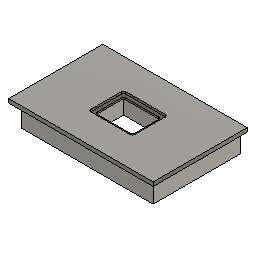
Freestafel - v1 v6 (Autodesk Fusion 360 design; units mm, degrees)
Autodesk Fusion 360 part; units mm, degrees
sketch "Sketch1" plane through (0, 0, 0) normal (0, 0, 1) x (1, 0, 0) in component "Freesblad"
  line L0 (0, 0) -> (660, 0)
  line L1 (660, 0) -> (660, 430)
  line L2 (660, 430) -> (0, 430)
  line L3 (0, 430) -> (0, 0)
  dimension "d10" = 660
  dimension "d11" = 430
  constraint horizontal L0
  constraint vertical L1
  constraint horizontal L2
  constraint vertical L3
  constraint coincident L0.start L3.end
  measures "d10" distance of L0.start L0.end
  measures "d11" distance of L0.start L2.end
extrude "Extrude1" add sketch "Sketch1" along normal blind 18 makes body 1 in component "Freesblad"
sketch "Sketch2" plane through (0, 0, 18) normal (0, 0, 1) x (-1, 0, 0) in component "Freesblad"
  line L0 (0, -430) -> (0, 0)
  line L1 (0, 0) -> (-660, 0)
  line L2 (-660, 0) -> (-660, -430)
  line L3 (-660, -430) -> (0, -430)
  line L4 (-420, -135) -> (-240, -135)
  line L5 (-230, -145) -> (-230, -285)
  line L6 (-240, -295) -> (-420, -295)
  line L7 (-430, -285) -> (-430, -145)
  line L8 (-430, -135) -> (-230, -295) construction
  line L9 (-230, -135) -> (-430, -295) construction
  arc A0 (-430, -285) -> (-420, -295) centre (-420, -285) ccw
  arc A1 (-240, -295) -> (-230, -285) centre (-240, -285) ccw
  arc A2 (-230, -145) -> (-240, -135) centre (-240, -145) ccw
  arc A3 (-420, -135) -> (-430, -145) centre (-420, -145) ccw
  arc A4 (-450, -285) -> (-420, -315) centre (-420, -285) ccw
  line L10 (-240, -315) -> (-420, -315)
  arc A5 (-240, -315) -> (-210, -285) centre (-240, -285) ccw
  line L11 (-210, -145) -> (-210, -285)
  arc A6 (-210, -145) -> (-240, -115) centre (-240, -145) ccw
  line L12 (-420, -115) -> (-240, -115)
  arc A7 (-420, -115) -> (-450, -145) centre (-420, -145) ccw
  line L13 (-450, -285) -> (-450, -145)
  point P0 (-330, -215)
  dimension "d16" = 200
  dimension "d17" = 160
  dimension "d18" = 10
  dimension "d19" = 10
  dimension "d20" = 10
  dimension "d21" = 10
  dimension "d40" = 215
  dimension "d41" = 330
  dimension "d42" = -20
  constraint horizontal L4
  constraint perpendicular L4 L5
  constraint parallel L4 L6
  constraint parallel L5 L7
  constraint coincident L8 P0
  constraint coincident L9 P0
  constraint coincident L9.end L6
  constraint coincident L9.end L7
  constraint tangent L6 A0
  constraint tangent L7 A0
  constraint coincident L8.end L5
  constraint coincident L8.end L6
  constraint tangent L5 A1
  constraint tangent L6 A1
  constraint coincident L9.start L5
  constraint coincident L9.start L4
  constraint tangent L5 A2
  constraint tangent L4 A2
  constraint coincident L8.start L7
  constraint coincident L8.start L4
  constraint tangent L7 A3
  constraint tangent L4 A3
  measures "d16" distance of L8.end L9.end
  measures "d17" distance of L9.start L8.end
  measures "d18" radius of A0
  measures "d19" radius of A1
  measures "d20" radius of A2
  measures "d21" radius of A3
  measures "d40" distance of L1 P0
  measures "d41" distance of L0 P0
  measures "d42" distance of A0
extrude "Extrude2" cut sketch "Sketch2" against normal blind 10 contours L4 L5 L6 L7 A0 A1 A2 A3 bodies 1 in component "Freesblad"
sketch "Sketch4" plane through (0, 0, 8) normal (0, 0, 1) x (-1, 0, 0) in component "Freesblad"
  arc A0 (-230, -145) -> (-240, -135) centre (-240, -145) ccw
  line L0 (-240, -135) -> (-420, -135)
  arc A1 (-420, -135) -> (-430, -145) centre (-420, -145) ccw
  line L1 (-430, -145) -> (-430, -285)
  arc A2 (-430, -285) -> (-420, -295) centre (-420, -285) ccw
  line L2 (-420, -295) -> (-240, -295)
  arc A3 (-240, -295) -> (-230, -285) centre (-240, -285) ccw
  line L3 (-230, -285) -> (-230, -145)
  line L4 (-245, -270) -> (-245, -160)
  line L5 (-255, -150) -> (-405, -150)
  line L6 (-415, -160) -> (-415, -270)
  line L7 (-405, -280) -> (-255, -280)
  arc A4 (-255, -280) -> (-245, -270) centre (-255, -270) ccw
  arc A5 (-415, -270) -> (-405, -280) centre (-405, -270) ccw
  arc A6 (-245, -160) -> (-255, -150) centre (-255, -160) ccw
  arc A7 (-405, -150) -> (-415, -160) centre (-405, -160) ccw
  dimension "d34" = 10
  dimension "d35" = 10
  dimension "d36" = 10
  dimension "d37" = 10
  constraint tangent L7 A4
  constraint tangent L4 A4
  constraint tangent L7 A5
  constraint tangent L6 A5
  constraint tangent L4 A6
  constraint tangent L5 A6
  constraint tangent L5 A7
  constraint tangent L6 A7
  measures "d19" radius of A6.centre
  measures "d20" radius of A6.centre
  measures "d34" radius of A4
  measures "d35" radius of A5
  measures "d36" radius of A6
  measures "d37" radius of A7
  measures "d43" distance of A6.centre
extrude "Extrude4" cut sketch "Sketch4" against normal blind 8 contours L4 L5 L6 L7 A4 A5 A6 A7 bodies 1 in component "Freesblad"
sketch "Sketch3" plane through (0, 0, 0) normal (0, 0, 1) x (1, 0, 0) in component "Freesblad"
  line L0 (30, 30) -> (630, 30)
  line L1 (630, 30) -> (630, 430)
  line L2 (630, 430) -> (30, 430)
  line L3 (30, 430) -> (30, 30)
  line L4 (48, 48) -> (612, 48)
  line L5 (612, 48) -> (612, 412)
  line L6 (612, 412) -> (48, 412)
  line L7 (48, 412) -> (48, 48)
  dimension "d24" = 600
  dimension "d25" = 400
  dimension "d28" = 30
  dimension "d29" = 30
  constraint horizontal L0
  constraint vertical L1
  constraint horizontal L2
  constraint vertical L3
  measures "d24" distance of L0.start L0.end
  measures "d25" distance of L0.start L2.end
  measures "d28" vertical distance of origin L0.start
  measures "d29" horizontal distance of origin L0.start
extrude "Extrude3" add sketch "Sketch3" against normal blind 100 separate body makes body 2 in component "Freesblad"
sketch "Sketch5" plane through (0, 0, 0) normal (0, 0, 1) x (-1, 0, 0) in component "Freesblad"
  line L0 (-48, -48) -> (-48, -412)
  line L1 (-48, -412) -> (-612, -412)
  line L2 (-612, -412) -> (-612, -48)
  line L3 (-612, -48) -> (-48, -48)
  line L4 (-30, -430) -> (-30, -30)
  line L5 (-30, -30) -> (-630, -30)
  line L6 (-630, -30) -> (-630, -430)
  line L7 (-630, -430) -> (-30, -430)
  line L8 (-210, -145) -> (-210, -285)
  line L9 (-240, -315) -> (-420, -315)
  line L10 (-450, -285) -> (-450, -145)
  line L11 (-420, -115) -> (-240, -115)
  line L12 (-210, -412) -> (-192, -412)
  line L13 (-192, -412) -> (-192, -48)
  line L14 (-192, -48) -> (-210, -48)
  line L15 (-210, -48) -> (-210, -412)
  line L16 (-450, -412) -> (-468, -412)
  line L17 (-468, -412) -> (-468, -48)
  line L18 (-468, -48) -> (-450, -48)
  line L19 (-450, -48) -> (-450, -412)
  line L20 (-48, -315) -> (-612, -315)
  line L21 (-612, -315) -> (-612, -333)
  line L22 (-612, -333) -> (-48, -333)
  line L23 (-48, -333) -> (-48, -315)
  line L24 (-48, -115) -> (-612, -115)
  line L25 (-612, -115) -> (-612, -97)
  line L26 (-612, -97) -> (-48, -97)
  line L27 (-48, -97) -> (-48, -115)
  dimension "d43" = 18
  dimension "d44" = 18
  dimension "d45" = 18
  dimension "d46" = 18
  constraint horizontal L12
  constraint vertical L13
  constraint horizontal L14
  constraint vertical L15
  constraint coincident L3 L13.end
  constraint coincident L1 L12.start
  constraint horizontal L16
  constraint vertical L17
  constraint horizontal L18
  constraint vertical L19
  constraint coincident L3 L17.end
  constraint coincident L1 L16.start
  constraint horizontal L20
  constraint vertical L21
  constraint horizontal L22
  constraint vertical L23
  constraint coincident L2 L21.end
  constraint coincident L0 L20.start
  constraint horizontal L24
  constraint vertical L25
  constraint horizontal L26
  constraint vertical L27
  constraint coincident L2 L25.end
  constraint coincident L0 L24.start
  constraint collinear L9 L20
  constraint collinear L11 L24
  constraint collinear L8 L15
  constraint collinear L10 L19
  measures "d43" distance of L12.start L12.end
  measures "d44" distance of L16.start L16.end
  measures "d45" distance of L20.start L22.end
  measures "d46" distance of L24.start L26.end
extrude "Extrude5" add sketch "Sketch5" against normal blind 100 separate body contours L0 L13 L24 L26 L27 | L0 L13 L20 L22 L23 | L11 L15 L19 L24 L26 | L9 L15 L19 L20 L22 | L2 L17 L24 L25 L26 | L2 L17 L20 L21 L22 makes body 3 at (144, 97, -33.3333) makes body 4 at (144, 333, -33.3333) makes body 5 at (290, 115, -33.3333) makes body 6 at (564, 333, -33.3333) makes body 7 at (370, 333, -33.3333) makes body 8 at (564, 97, -33.3333) in component "Freesblad"
extrude "Extrude6" add sketch "Sketch5" against normal blind 50 contours L13 L15 L24 L26 | L13 L15 L20 L22 | L17 L19 L24 L26 | L17 L19 L20 L22 bodies 3 4 5 6 7 8 in component "Freesblad"
extrude "Extrude7" add sketch "Sketch5" against normal blind 100 separate body contours L3 L13 L14 L15 L26 | L13 L15 L24 L26 | L8 L13 L15 L20 L24 | L3 L17 L18 L19 L26 | L13 L15 L20 L22 | L17 L19 L24 L26 | L1 L12 L13 L15 L22 | L10 L17 L19 L20 L24 | L17 L19 L20 L22 | L1 L16 L17 L19 L22 makes body 9 at (192, 290.6667, -33.3333) makes body 10 at (468, 290.6667, -33.3333) in component "Freesblad"
extrude "Extrude8" cut sketch "Sketch5" against normal blind 50 contours L13 L15 L24 L26 | L13 L15 L20 L22 | L17 L19 L24 L26 | L17 L19 L20 L22 bodies 9 10 in component "Freesblad"
sketch "Haaklat" plane through (630, 0, 0) normal (1, 0, 0) x (0, 1, 0) in component "Freesblad"
  line L0 (430, 0) -> (30, 0)
  line L1 (30, 0) -> (30, -100)
  line L2 (30, -100) -> (430, -100)
  line L3 (430, -100) -> (430, 0)
  line L4 (430, 0) -> (448, 0)
  line L5 (448, 0) -> (448, -45)
  line L6 (430, -27) -> (430, 0)
  line L7 (448, -45) -> (430, -27)
  dimension "d55" = 18
  dimension "d58" = 45
  dimension "d59" = 45
  constraint horizontal L4
  constraint vertical L5
  constraint vertical L6
  constraint coincident L0.start L3.end
  measures "d55" distance of L0.start L4.end
  measures "d58" angle of L5 L7
  measures "d59" distance of L4.end L5.end
extrude "Extrude9" add sketch "Haaklat" against normal blind 600 separate body contours L3 L4 L5 L6 L7 makes body 11 in component "Freesblad"
component "Freesblad" placed x (1, 0, 0) y (0, 1, 0) z (0, 0, 1) at (0, 0, 0)
hidden bodies 11
equation "mod_breedte = 600 mm"
equation "mod_diepte = 400 mm"
equation "blad_overstek = 30 mm"
equation "blad_dikte = 18 mm"
equation "torsionbox_hoogte = 100 mm"
equation "inlegplaat_breedte = 200 mm"
equation "inlegplaat_diepte = 160 mm"
equation "inlegplaat_dikte = 10 mm"
equation "inlegplaat_hoekradius = 10 mm"
equation "d10 = mod_breedte + ( 2 * blad_overstek )"
equation "d11 = mod_diepte + blad_overstek"
equation "d12 = blad_dikte"
equation "inlegplaat_center_offset = 215 mm"
equation "d16 = inlegplaat_breedte"
equation "d17 = inlegplaat_diepte"
equation "d18 = inlegplaat_hoekradius"
equation "d19 = inlegplaat_hoekradius"
equation "d20 = inlegplaat_hoekradius"
equation "d21 = inlegplaat_hoekradius"
equation "d22 = -1 * inlegplaat_dikte"
equation "d24 = mod_breedte"
equation "d25 = mod_diepte"
equation "torsionbox_dikte = 18 mm"
equation "d27 = -torsionbox_dikte"
equation "d28 = blad_overstek"
equation "d29 = blad_overstek"
equation "d30 = -mod_hoogte"
equation "d34 = inlegplaat_hoekradius"
equation "d35 = inlegplaat_hoekradius"
equation "d36 = inlegplaat_hoekradius"
equation "d37 = inlegplaat_hoekradius"
equation "d38 = -blad_dikte + inlegplaat_dikte"
equation "d40 = inlegplaat_center_offset"
equation "d41 = ( mod_breedte + ( 2 * blad_overstek ) ) / 2"
equation "d47 = -torsionbox_hoogte"
equation "d49 = torsionbox_hoogte / -2"
equation "d51 = -torsionbox_hoogte"
equation "d53 = torsionbox_hoogte / -2"
equation "d60 = -mod_breedte"
equation "mod_hoogte = 100 mm"
named bodies: "Blad", "Module", "Torsion3", "Torsion4", "Torsion1", "Torsion2", "Haaklat"
